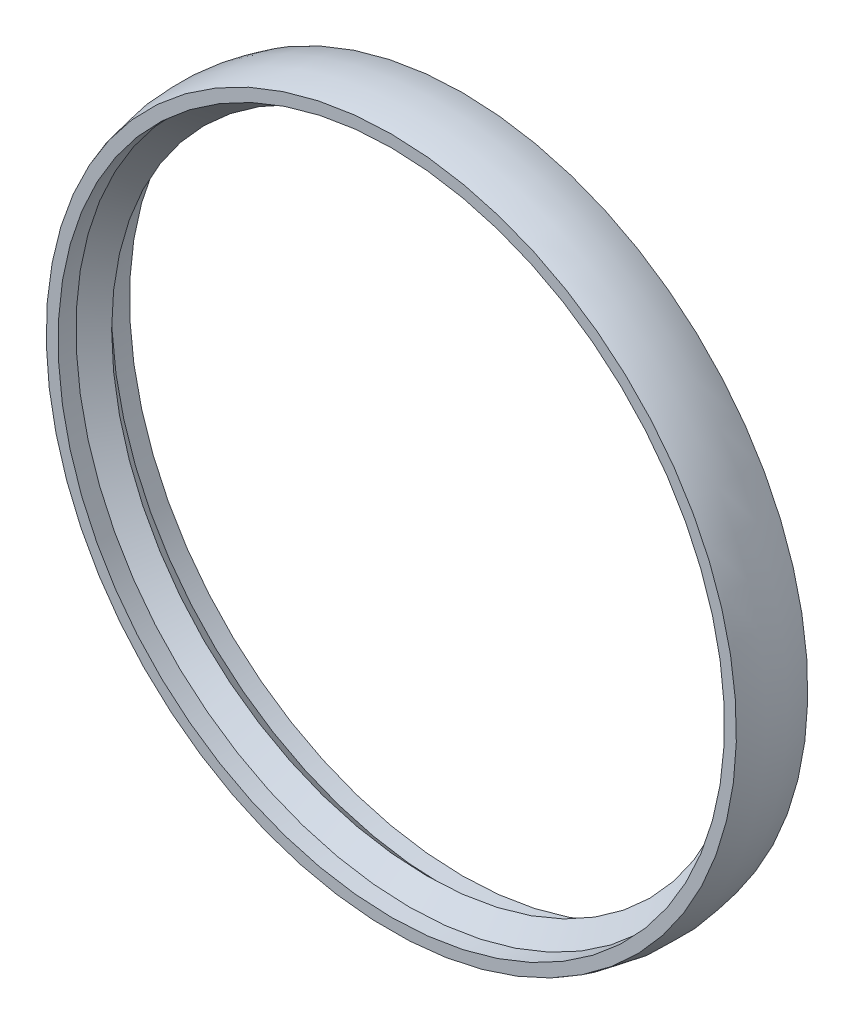
# Autodesk Inventor part: tyre
Saved by Autodesk Inventor 2018 (Build 220112000, 112)
## iProperties
Created: 2017-10-30
Part Number: tyre
Material: Generic
Document SubType Name: Modeling
Designer: erwin
Density: 1 g/cm^3
Appearance: Default
Author: erwin
Autodesk Inventor part; units mm, degrees
ref_plane "YZ Plane" through (0, 0, 0) normal (1, 0, 0) x (0, 1, 0)
ref_plane "XZ Plane" through (0, 0, 0) normal (0, 1, 0) x (-1, 0, 0)
ref_plane "XY Plane" through (0, 0, 0) normal (0, 0, 1) x (1, 0, 0)
sketch "Sketch2" plane through (0, 0, 0) normal (1, 0, 0) x (0, 1, 0)
  line L0 (26, 0) -> (26, -1.3929)
  line L1 (26, -1.3929) -> (24.6071, -2.7857)
  line L2 (24.6071, -2.7857) -> (26, -4.1786)
  line L3 (26, -4.1786) -> (26, -5.5714)
  line L4 (26, 0) -> (26.9286, 0)
  line L5 (26.9286, -5.5714) -> (26, -5.5714)
  arc A0 (26.9286, -5.5714) -> (26.9286, 0) centre (18.0706, -2.7857) ccw
  line L6 (26, -5.5714) -> (26, -4.1786)
  line L7 (26, -1.3929) -> (26, 0)
  line L8 (0, 0) -> (0, -17.6921) construction
  dimension "d2" = 26
  constraints: 18 end point, 2 point on circle, 1 centre point, 1 vertical
  measures "d2" distance between parallel lines of L8 L0
revolve "Revolution1" add sketch "Sketch2" angle 360 about axis through (0, 0, 0) along (0, 0, -1)
body "Solid1"
